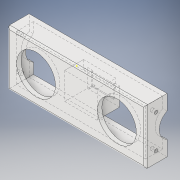
# Autodesk Inventor part: Baseplate
Saved by Autodesk Inventor 2019 (Build 230136000, 136)
## iProperties
Created: 2018-12-23
Part Number: Baseplate
Material: Generic
Document SubType Name: Modeling
Designer: Martin
Density: 1 g/cm^3
Appearance: Default
Author: Martin
Autodesk Inventor part; units mm, degrees
ref_plane "YZ Plane" through (0, 0, 0) normal (1, 0, 0) x (0, 1, 0)
ref_plane "XZ Plane" through (0, 0, 0) normal (0, 1, 0) x (-1, 0, 0)
ref_plane "XY Plane" through (0, 0, 0) normal (0, 0, 1) x (1, 0, 0)
sketch "Sketch2" plane through (0, 0, 0) normal (0, 0, 1) x (1, 0, 0)
  line L0 (-60, 21.25) -> (60, 21.25)
  line L1 (60, 21.25) -> (60, -21.25)
  line L2 (60, -21.25) -> (-60, -21.25)
  line L3 (-60, -21.25) -> (-60, 21.25)
  line L4 (-60, 21.25) -> (60, -21.25) construction
  line L5 (60, 21.25) -> (-60, -21.25) construction
  line L6 (-64, 25.5) -> (64, 25.5)
  line L7 (64, 25.5) -> (64, -25.5)
  line L8 (64, -25.5) -> (-64, -25.5)
  line L9 (-64, -25.5) -> (-64, 25.5)
  line L10 (-64, 25.5) -> (64, -25.5) construction
  line L11 (64, 25.5) -> (-64, -25.5) construction
  line L12 (-15, 12.5) -> (15, 12.5)
  line L13 (15, 12.5) -> (15, -12.5)
  line L14 (15, -12.5) -> (-15, -12.5)
  line L15 (-15, -12.5) -> (-15, 12.5)
  line L16 (-15, 12.5) -> (15, -12.5) construction
  line L17 (15, 12.5) -> (-15, -12.5) construction
  circle A0 centre (37.5, 0) radius 18
  circle A1 centre (-37.5, 0) radius 18
  point P0 (0, 0)
  point P1 (0, 0)
  dimension "d0" = 120
  dimension "d1" = 42.5
  dimension "d2" = 60
  dimension "d3" = 21.25
  dimension "d4" = 128
  dimension "d5" = 51
  dimension "d28" = 30
  dimension "d29" = 25
  dimension "d32" = 45
  dimension "d33" = 36
  dimension "d34" = 22.5
  dimension "d35" = 45
  dimension "d36" = 36
  dimension "d37" = 22.5
  dimension "d38" = 21.25
  dimension "d39" = 21.25
  constraints: 36 end point, 6 midpoint, 6 parallel, 3 horizontal, 3 perpendicular, 2 centre point
  measures "d0" distance of L0.start L0.end
  measures "d1" distance of L2.end L0.start
  measures "d2" distance from line of point (0, 0) L3
  measures "d3" distance from line of point (0, 0) L2
  measures "d4" distance of L7.end L8.end
  measures "d5" distance of L6.end L7.end
  measures "d28" distance of L12.start L12.end
  measures "d29" distance of L12.end L13.end
  measures "d32" distance between parallel lines of L13 L1
  measures "d33" diameter of A0
  measures "d34" distance from line of A0.centre L1
  measures "d35" distance between parallel lines of L15 L3
  measures "d36" diameter of A1
  measures "d37" distance from line of L3 A1.centre
  measures "d38" distance from line of L2 A1.centre
  measures "d39" distance from line of L2 A0.centre
extrude "Extrusion1" add sketch "Sketch2" against normal blind 4 contours L0 L1 L2 L3 | L12 L13 L14 L15 | A0 | A1
extrude "Extrusion2" add sketch "Sketch2" against normal blind 20 contours L6 L7 L8 L9
fillet "Fillet1" radius 2 4 edges at (-64, 0, 0) (0, 25.5, 0) (64, 0, 0) (0, -25.5, 0)
sketch "Sketch3" plane through (-64, -25.5, -20) normal (-1, 0, 0) x (0, 0, 1)
  line L0 (16, 4.25) -> (16, 46.75) projected
  line L1 (16, 4.25) -> (-26.5, 4.25)
  line L2 (-26.5, 4.25) -> (-26.5, 46.75)
  line L3 (-26.5, 46.75) -> (16, 46.75)
  line L4 (16, 46.75) -> (16, 4.25)
  circle A0 centre (-5.25, 25.5) radius 11 construction
  circle A1 centre (-5.25, 25.5) radius 12.5
  circle A2 centre (10.25, 10) radius 1.5
  circle A3 centre (10.25, 41) radius 1.5
  point P0 (20, 25.5)
  dimension "d11" = 42.5
  dimension "d12" = 22
  dimension "d13" = 25
  dimension "d16" = 3
  dimension "d17" = 3
  dimension "d19" = 15.5
  dimension "d20" = 21.25
  dimension "d21" = 42.5
  dimension "d22" = 21.25
  dimension "d23" = 15.5
  dimension "d24" = 15.5
  dimension "d25" = 15.5
  constraints: 8 end point, 4 centre point, 2 parallel, 1 coincident, 1 horizontal, 1 perpendicular
  measures "d11" distance of L2.end L3.end
  measures "d12" diameter of A0
  measures "d13" diameter of A1
  measures "d16" diameter of A2
  measures "d17" diameter of A3
  measures "d19" horizontal distance of A2.centre A0.centre
  measures "d20" distance from line of A0.centre L1
  measures "d21" distance between parallel lines of L3 L1
  measures "d22" distance from line of L0 A0.centre
  measures "d23" horizontal distance of A2.centre A0.centre
  measures "d24" horizontal distance of A3.centre A0.centre
  measures "d25" horizontal distance of A3.centre A0.centre
extrude "Extrusion3" cut sketch "Sketch3" against normal blind 150 contours A1
sketch "Sketch5" plane through (-64, 25.5, -20) normal (0, 1, 0) x (1, 0, 0)
  point P0 (64, -20)
extrude "Extrusion4" cut sketch "Sketch3" against normal blind 150 contours A2 | A3
extrude "Extrusion5" add sketch "Sketch2" against normal blind 24 contours L12 L13 L14 L15
extrude "Extrusion6" cut sketch "Sketch2" against normal blind 24 contours A0 | A1
sketch "Sketch6" plane through (0, 0, -24) normal (0, 0, -1) x (-1, 0, 0)
  line L0 (-10.3, 8) -> (10.3, 8)
  line L1 (10.3, 8) -> (10.3, -8)
  line L2 (10.3, -8) -> (-10.3, -8)
  line L3 (-10.3, -8) -> (-10.3, 8)
  line L4 (-10.3, 8) -> (10.3, -8) construction
  line L5 (10.3, 8) -> (-10.3, -8) construction
  line L6 (-15, -12.5) -> (-15, 12.5) projected
  line L7 (15, -12.5) -> (-15, -12.5) projected
  line L8 (-15, 12.5) -> (15, 12.5)
  line L9 (15, 12.5) -> (15, -12.5)
  line L10 (15, -12.5) -> (-15, -12.5)
  line L11 (-15, -12.5) -> (-15, 12.5)
  line L12 (15, 12.5) -> (15, -12.5) projected
  line L13 (-15, 12.5) -> (15, 12.5)
  line L14 (15, 12.5) -> (15, 4.5)
  line L15 (15, 4.5) -> (-15, 4.5)
  line L16 (-15, 4.5) -> (-15, 12.5)
  point P0 (0, 0)
  dimension "d42" = 20.6
  dimension "d43" = 16
  dimension "d46" = 12.5
  constraints: 28 end point, 6 parallel, 3 horizontal, 3 perpendicular, 2 midpoint, 1 point on line
  measures "d42" distance of L1.end L2.end
  measures "d43" distance of L0.end L1.end
  measures "d46" distance between parallel lines of L2 L15
extrude "Extrusion7" add sketch "Sketch6" along normal blind 1 contours L3 L15 L6 L8 L9 L1 L0 | L3 L2 L1 L15 L9 L7 L6
extrude "Extrusion8" cut sketch "Sketch6" along normal mid plane 5 contours L3 L15 L6 L8 L9 L1 L0 | L0 L1 L15 L3
sketch "Sketch7" plane through (0, 0, -24) normal (0, 0, -1) x (-1, 0, 0)
  line L0 (10.3, -8) -> (-10.3, -8) projected
  line L1 (10.3, 4.5) -> (-10.3, 4.5) projected
  line L2 (10.3, -8) -> (-10.3, -8)
  line L3 (-10.3, -8) -> (-10.3, 4.5)
  line L4 (-10.3, 4.5) -> (10.3, 4.5)
  line L5 (10.3, 4.5) -> (10.3, -8)
  circle A0 centre (7.3, -5.55) radius 0.5
  circle A1 centre (-7.3, -5.55) radius 0.5
  point P0 (0, 0)
  dimension "d49" = 1
  dimension "d50" = 1
  dimension "d51" = 3
  dimension "d52" = 3
  dimension "d53" = 2.45
  dimension "d54" = 2.45
  dimension "d55" = 14.6
  constraints: 8 end point, 2 centre point, 2 parallel, 1 horizontal, 1 perpendicular
  measures "d49" diameter of A0
  measures "d50" diameter of A1
  measures "d51" distance from line of L5 A0.centre
  measures "d52" distance from line of L3 A1.centre
  measures "d53" distance from line of A0.centre L0
  measures "d54" distance from line of A1.centre L0
  measures "d55" distance of A1.centre A0.centre
extrude "Extrusion9" cut sketch "Sketch7" against normal blind 5 contours A0 | A1
equation "\"d2\" = 0.5 * d0"
equation "\"d3\" = 0.5 * d1"
equation "\"d34\" = 0.5 * d32"
equation "\"d37\" = 0.5 * d35"
equation "\"d38\" = 0.5 * d1"
equation "\"d39\" = 0.5 * d1"
equation "\"d20\" = 0.5 * d21"
equation "\"d21\" = d11"
equation "\"d22\" = 0.5 * d11"
equation "\"d52\" = d51"
equation "\"d54\" = d53"
body "Solid1"
